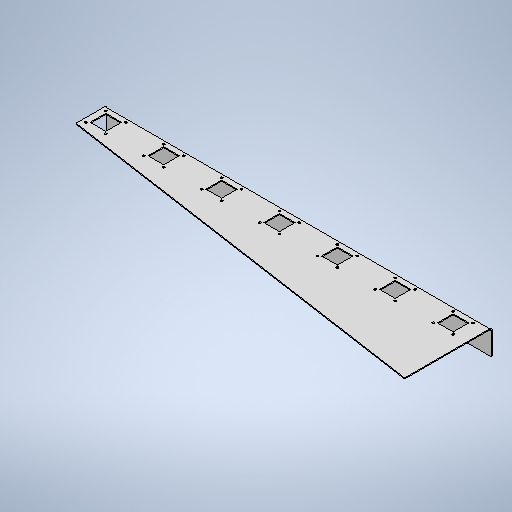
# Autodesk Inventor part: TKS 3005 BOTTOM DS diameter way
Saved by Autodesk Inventor 2025 (Build 290162010, 162A)
## iProperties
Created: 2024-12-09
Part Number: TKS 3005 BOTTOM DS diameter way
Material: Stainless Steel
Document SubType Name: Sheet Metal
Designer: user
Mass: 3269.02 g
Surface Area: 1007.63 cm^2
Volume: 408.627 cm^3
Density: 8 g/cm^3
Flat Pattern Width: 35.3927 cm
Flat Pattern Length: 123 cm
Flat Pattern Area: 4353.31 cm^2
Sheet Metal Rule: AISI304 3mm Die 32
Sheet Metal Width: 353,927 mm
Sheet Metal Length: 1230,000 mm
Sheet Metal Area: 435330,742 mm^2
Appearance: Default
Author: user
Autodesk Inventor part; units mm, degrees
ref_plane "YZ Plane" through (0, 0, 0) normal (1, 0, 0) x (0, 1, 0)
ref_plane "XZ Plane" through (0, 0, 0) normal (0, 1, 0) x (-1, 0, 0)
ref_plane "XY Plane" through (0, 0, 0) normal (0, 0, 1) x (1, 0, 0)
sketch "Sketch1" plane through (0, 0, 0) normal (0, 0, 1) x (1, 0, 0)
  line L0 (700, 140) -> (-700, 140)
  line L1 (-700, 140) -> (-700, -140)
  line L2 (-700, -140) -> (700, -140)
  line L3 (700, -140) -> (700, 140)
  line L4 (700, 140) -> (-700, -140) construction
  line L5 (-700, 140) -> (700, -140) construction
  line L6 (-530, 140) -> (-530, 40)
  line L7 (-530, 40) -> (700, -140)
  point P0 (0, 0)
  point P1 (0, 0)
  point P2 (700, 0)
  dimension "d32" = 280
  dimension "d33" = 1400
  dimension "d60" = 100
  dimension "d61" = 1230
  measures "d32" distance of L2.end L0.start
  measures "d33" distance of L1.end L2.end
  measures "d60" distance of L6.start L6.end
  measures "d61" distance between parallel lines of L3 L6
extrude "Plate1" add sketch "Sketch1" along normal blind 3 contours L3 L7 L6 L0
sketch "Sketch8" plane through (0, 0, 3) normal (0, 0, 1) x (1, 0, 0)
  line L0 (650, 65) -> (600, 65)
  line L1 (600, 65) -> (600, 115)
  line L2 (600, 115) -> (650, 115)
  line L3 (650, 115) -> (650, 65)
  line L4 (650, 65) -> (600, 115) construction
  line L5 (600, 65) -> (650, 115) construction
  circle A0 centre (656.8198, 58.1802) radius 3.5
  circle A1 centre (593.1802, 58.1802) radius 3.5
  circle A2 centre (593.1802, 121.8198) radius 3.5
  circle A3 centre (656.8198, 121.8198) radius 3.5
  circle A4 centre (625, 90) radius 45 construction
  line L6 (700, 140) -> (700, -140) projected
  line L7 (-530, 140) -> (700, 140) projected
  point P0 (0, 0)
  dimension "d51" = 50
  dimension "d52" = 50
  dimension "d53" = 7
  dimension "d54" = 90
  dimension "d72" = 75
  dimension "d73" = 50
  constraints: 12 end point, 5 centre point, 4 point on circle, 4 point on line, 3 equal radius, 2 midpoint, 2 parallel, 1 coincident, 1 horizontal, 1 perpendicular
  measures "d51" distance of L0.start L0.end
  measures "d52" distance of L0.end L1.end
  measures "d53" diameter of A0
  measures "d54" diameter of A4
  measures "d72" distance from line of L6 point (625, 90)
  measures "d73" distance from line of point (625, 90) L7
extrude "Cut3" cut sketch "Sketch8" against normal blind 3
pattern_linear "Rectangular Pattern1" count 7 spacing 185 along (-1, 0, 0) of "Cut3"
sketch "Sketch9" plane through (700, 137, 3) normal (0, 1, 0) x (-1, 0, 0)
  line L0 (1230, 0) -> (0, 0)
  line L1 (0, 0) -> (0, -80)
  line L2 (0, -80) -> (1230, -80)
  line L3 (1230, -80) -> (1230, 0)
  constraints: 6 end point, 1 horizontal, 1 perpendicular, 1 vertical
edge flange "Flange3" height 80 angle 90 thickness 3 bend radius 5 thickness toward (0, 1, 0) relief round relief width 3 relief depth 1.5 edges at (85, 140, 0) wall of the first edge with corners at (-530, 137, 3) (700, 137, 3) (700, 137, -77) (-530, 137, -77)
bend "Bend3"
corner "Corner3"
equation "\"d55\" = Thickness"
equation "\"d2\" = Thickness"
equation "\"d62\" = BendReliefWidth"
equation "\"d63\" = BendReliefDepth"
equation "\"d64\" = MinimumRemnant"
equation "\"d65\" = TransitionRadius"
equation "\"d68\" = BendRadius"
equation "\"d69\" = CornerReliefSize"
equation "\"d70\" = GapSize"
equation "\"d71\" = JacobiRadiusSize"
equation "\"BendReliefWidth\" = Thickness"
equation "\"BendReliefDepth\" = 0.5 * Thickness"
equation "\"CornerReliefSize\" = 4 * Thickness"
equation "\"MinimumRemnant\" = 2 * Thickness"
equation "\"TransitionRadius\" = BendRadius"
equation "\"JacobiRadiusSize\" = BendRadius"
equation "\"GapSize\" = Thickness"
equation "\"Thickness\" = 3"
equation "\"BendRadius\" = 5"
body "Solid1"
